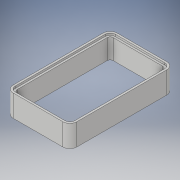
# Autodesk Inventor part: cover
Saved by Autodesk Inventor 2019 (Build 230136000, 136)
## iProperties
Created: 2022-02-05
Part Number: cover
Material: Generic
Document SubType Name: Modeling
Designer: josec
Density: 1 g/cm^3
Appearance: Default
Author: josec
Autodesk Inventor part; units mm, degrees
ref_plane "YZ Plane" through (0, 0, 0) normal (1, 0, 0) x (0, 1, 0)
ref_plane "XZ Plane" through (0, 0, 0) normal (0, 1, 0) x (-1, 0, 0)
ref_plane "XY Plane" through (0, 0, 0) normal (0, 0, 1) x (1, 0, 0)
sketch "Sketch1" plane through (0, 0, 0) normal (0, 1, 0) x (-1, 0, 0)
  line L0 (-5, 0) -> (-55, 0)
  line L1 (-60, -5) -> (-60, -95.5)
  line L2 (-55, -100.5) -> (-5, -100.5)
  line L3 (0, -95.5) -> (0, -5)
  arc A0 (-5, -100.5) -> (0, -95.5) centre (-5, -95.5) ccw
  arc A1 (-60, -95.5) -> (-55, -100.5) centre (-55, -95.5) ccw
  arc A2 (-55, 0) -> (-60, -5) centre (-55, -5) ccw
  arc A3 (0, -5) -> (-5, 0) centre (-5, -5) ccw
  line L4 (-62, -95.5) -> (-62, -5)
  arc A4 (-55, 2) -> (-62, -5) centre (-55, -5) ccw
  line L5 (-55, 2) -> (-5, 2)
  arc A5 (2, -5) -> (-5, 2) centre (-5, -5) ccw
  line L6 (2, -5) -> (2, -95.5)
  arc A6 (-5, -102.5) -> (2, -95.5) centre (-5, -95.5) ccw
  line L7 (-5, -102.5) -> (-55, -102.5)
  arc A7 (-62, -95.5) -> (-55, -102.5) centre (-55, -95.5) ccw
  point P0 (0, 0)
  point P1 (-60, -100.5)
  point P2 (-60, 0)
  point P3 (0, -100.5)
  dimension "d0" = 60
  dimension "d1" = 100.5
  dimension "d2" = 5
  dimension "d3" = 2
  constraints: 16 end point, 16 point on circle, 8 centre point, 8 point on line, 8 tangent, 4 parallel, 3 equal radius, 2 perpendicular, 1 horizontal, 7 other
  measures "d0" distance of point (0, -100.5) point (-60, -100.5)
  measures "d1" distance of point (-60, -100.5) point (-60, 0)
  measures "d2" radius of A0
  measures "d3" distance between parallel lines of L1 L4
extrude "Extrusion1" add sketch "Sketch1" along normal blind 22
sketch "Sketch3" plane through (0, 0, 0) normal (0, -1, 0) x (1, 0, 0)
  line L0 (5, 0) -> (55, 0)
  line L1 (60, -5) -> (60, -95.5)
  line L2 (55, -100.5) -> (5, -100.5)
  line L3 (0, -95.5) -> (0, -5)
  arc A0 (5, 0) -> (0, -5) centre (5, -5) ccw
  arc A1 (0, -95.5) -> (5, -100.5) centre (5, -95.5) ccw
  arc A2 (55, -100.5) -> (60, -95.5) centre (55, -95.5) ccw
  arc A3 (60, -5) -> (55, 0) centre (55, -5) ccw
  line L4 (2, -5) -> (2, -95.5)
  arc A4 (2, -95.5) -> (5, -98.5) centre (5, -95.5) ccw
  line L5 (5, -98.5) -> (55, -98.5)
  arc A5 (55, -98.5) -> (58, -95.5) centre (55, -95.5) ccw
  line L6 (58, -95.5) -> (58, -5)
  arc A6 (58, -5) -> (55, -2) centre (55, -5) ccw
  line L7 (55, -2) -> (5, -2)
  arc A7 (5, -2) -> (2, -5) centre (5, -5) ccw
  point P0 (0, 0)
  point P1 (60, -100.5)
  point P2 (60, 0)
  point P3 (0, -100.5)
  dimension "d12" = 60
  dimension "d13" = 100.5
  dimension "d14" = 5
  dimension "d15" = 2
  constraints: 16 end point, 16 point on circle, 8 centre point, 8 point on line, 8 tangent, 4 parallel, 3 equal radius, 2 perpendicular, 1 horizontal, 7 other
  measures "d12" distance of point (60, -100.5) point (0, -100.5)
  measures "d13" distance of point (60, 0) point (60, -100.5)
  measures "d14" radius of A0
  measures "d15" distance between parallel lines of L3 L4
extrude "Extrusion3" add sketch "Sketch3" against normal blind 20
body "Solid1"
